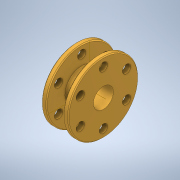
# Autodesk Inventor part: connecting rod hub
Saved by Autodesk Inventor 2021.1 (Build 251245000, 245)
## iProperties
Created: 2020-08-30
Part Number: connecting rod hub
Material: Brass, Soft Yellow
Document SubType Name: Sheet Metal
Designer: Vamshi
Mass: 1231.47 g
Surface Area: 428.954 cm^2
Volume: 145.392 cm^3
Density: 8.47 g/cm^3
Sheet Metal Rule: Default
Appearance: Brass - Satin
Author: Vamshi
Autodesk Inventor part; units mm, degrees
ref_plane "YZ Plane" through (0, 0, 0) normal (1, 0, 0) x (0, 1, 0)
ref_plane "XZ Plane" through (0, 0, 0) normal (0, 1, 0) x (-1, 0, 0)
ref_plane "XY Plane" through (0, 0, 0) normal (0, 0, 1) x (1, 0, 0)
sketch "Sketch1" plane through (0, 0, 0) normal (0, 0, 1) x (1, 0, 0)
  circle A0 centre (0, 0) radius 15.24
  circle A1 centre (0, 0) radius 25.4
  dimension "d0" = 30.48
  dimension "d1" = 50.8
  constraints: 2 centre point, 2 coincident
  measures "d0" diameter of A0
  measures "d1" diameter of A1
extrude "Extrusion1" add sketch "Sketch1" along normal mid plane 40.64
sketch "Sketch2" plane through (0, 0, 0) normal (1, 0, 0) x (0, 1, 0)
  line L0 (25.4, -20.32) -> (15.24, -20.32) projected
  line L1 (15.24, -20.32) -> (15.24, 20.32) projected
  line L2 (15.24, 20.32) -> (25.4, 20.32) projected
  line L3 (25.4, 20.32) -> (25.4, -20.32) projected
  line L4 (-15.24, -20.32) -> (-25.4, -20.32) projected
  line L5 (-25.4, -20.32) -> (-25.4, 20.32) projected
  line L6 (-25.4, 20.32) -> (-15.24, 20.32) projected
  line L7 (-15.24, 20.32) -> (-15.24, -20.32) projected
  line L8 (25.4, -20.32) -> (15.24, -20.32) projected
  line L9 (15.24, -20.32) -> (15.24, 20.32) projected
  line L10 (15.24, 20.32) -> (25.4, 20.32) projected
  line L11 (25.4, 20.32) -> (25.4, -20.32) projected
  line L12 (-15.24, -20.32) -> (-25.4, -20.32) projected
  line L13 (-25.4, -20.32) -> (-25.4, 20.32) projected
  line L14 (-25.4, 20.32) -> (-15.24, 20.32) projected
  line L15 (-15.24, 20.32) -> (-15.24, -20.32) projected
  line L16 (-25.4, -20.32) -> (25.4, -20.32) projected
  line L17 (25.4, 20.32) -> (-25.4, 20.32) projected
  line L18 (-25.4, -20.32) -> (-53.34, -20.32)
  line L19 (-53.34, -20.32) -> (-53.34, -12.7)
  line L20 (-53.34, -12.7) -> (-25.4, -12.7)
  line L21 (-25.4, -12.7) -> (-25.4, -20.32)
  line L22 (25.4, 20.32) -> (-25.4, 20.32) projected
  line L23 (-25.4, 20.32) -> (-53.34, 20.32)
  line L24 (-53.34, 20.32) -> (-53.34, 12.7)
  line L25 (-53.34, 12.7) -> (-25.4, 12.7)
  line L26 (-25.4, 12.7) -> (-25.4, 20.32)
  line L27 (0, -28.448) -> (0, 28.448) projected
  point P0 (0, 0)
  dimension "d4" = 27.94
  dimension "d5" = 7.62
  dimension "d6" = 27.94
  dimension "d7" = 7.62
  constraints: 16 end point, 4 parallel, 2 horizontal, 2 perpendicular
  measures "d4" distance of L19.end L20.end
  measures "d5" distance of L18.end L19.end
  measures "d6" distance of L25.end L24.end
  measures "d7" distance of L24.end L23.end
revolve "Revolution1" add sketch "Sketch2" angle 360 about axis through (0, 0, -10) along (0, 0, 1) contours L18 L19 L20 L5 | L5 L25 L24 L23
chamfer "Chamfer1" distance 1.27 angle 45 1 edges at (0, 53.34, -20.32) measured on face at (-31.6257, -42.9531, -15.24)
chamfer "Chamfer2" distance 1.27 angle 45 1 edges at (0, 53.34, -12.7) measured on face at (-31.6257, -42.9531, -14.8167)
chamfer "Chamfer3" distance 1.27 angle 45 2 edges at (0, 53.34, 20.32) (0, 53.34, 12.7) measured on face at (-31.6257, -42.9531, 17.78)
sketch "Sketch3" plane through (0, 0, 20.32) normal (0, 0, 1) x (1, 0, 0)
  circle A0 centre (0, 0) radius 40.64 construction
  circle A1 centre (0, 40.64) radius 6.35
  circle A2 centre (-35.1953, 20.32) radius 6.35
  circle A3 centre (-35.1953, -20.32) radius 6.35
  circle A4 centre (0, -40.64) radius 6.35
  circle A5 centre (35.1953, -20.32) radius 6.35
  circle A6 centre (35.1953, 20.32) radius 6.35
  dimension "d18" = 81.28
  dimension "d19" = 12.7
  dimension "d22" = 360
  constraints: 6 centre point, 1 coincident, 1 vertical alignment, 15 other
  measures "d19" diameter of A1
extrude "Extrusion2" cut sketch "Sketch3" against normal through all
equation "\"BendRadius\" = Thickness"
equation "\"BendReliefWidth\" = Thickness"
equation "\"BendReliefDepth\" = 0.5 * Thickness"
equation "\"CornerReliefSize\" = 4 * Thickness"
equation "\"MinimumRemnant\" = 2 * Thickness"
equation "\"TransitionRadius\" = BendRadius"
equation "\"JacobiRadiusSize\" = BendRadius"
equation "\"GapSize\" = Thickness"
equation "\"Thickness\" = 3.048"
body "Solid1"
